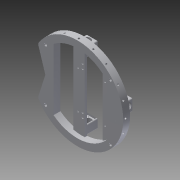
# Autodesk Inventor part: Middle Plate
Saved by Autodesk Inventor 2015 (Build 190159000, 159)
## iProperties
Created: 2015-10-10
Part Number: Middle Plate
Material: ABS Plastic
Document SubType Name: Modeling
Designer: James
Density: 1.06 g/cm^3
Appearance: Smooth - White
Author: James
Autodesk Inventor part; units mm, degrees
(part 1 of 2)
ref_plane "YZ Plane" through (0, 0, 0) normal (1, 0, 0) x (0, 1, 0)
ref_plane "XZ Plane" through (0, 0, 0) normal (0, 1, 0) x (-1, 0, 0)
ref_plane "XY Plane" through (0, 0, 0) normal (0, 0, 1) x (1, 0, 0)
sketch "Sketch1" plane through (0, 0, 0) normal (0, 1, 0) x (-1, 0, 0)
  line L0 (70, 0) -> (70, 48.2183)
  line L1 (70, 0) -> (70, -48.2183)
  arc A0 (70, 48.2183) -> (70, -48.2183) centre (0, 0) ccw
  arc A1 (85, 52.6783) -> (85, -52.6783) centre (0, 0) ccw
  line L2 (85, -52.6783) -> (85, -47.6783)
  line L3 (85, 52.6783) -> (85, 47.6783)
  line L4 (85, -47.6783) -> (70, 0)
  line L5 (70, 0) -> (85, 47.6783)
  dimension "d332" = 5
  dimension "d333" = 5
  constraints: 12 end point, 4 point on circle, 2 centre point, 1 coincident, 1 point on line, 1 vertical
  measures "d332" distance of L2.start L2.end
  measures "d333" distance of L3.start L3.end
extrude "Extrusion1" add sketch "Sketch1" along normal blind 15
sketch "Sketch2" plane through (0, 15, 0) normal (0, 1, 0) x (1, 0, 0)
  circle A0 centre (-69.5802, 56.8899) radius 3
  circle A1 centre (71.6532, 61.1111) radius 3
  circle A2 centre (-69.5802, -56.8899) radius 3
  circle A3 centre (71.6532, -61.1111) radius 3
  point P0 (0, 0)
  dimension "d10" = 6
  dimension "d11" = 6
  constraints: 4 centre point
  measures "d10" diameter of A0
  measures "d11" diameter of A1
extrude "Extrusion2" cut sketch "Sketch2" against normal blind 15
sketch "Sketch3" plane through (0, 15, 0) normal (0, 1, 0) x (1, 0, 0)
  line L0 (-85, 52.6783) -> (-85, -52.6783) projected
  line L1 (-62, 5.2) -> (-62, -5.2)
  line L2 (-62, -5.2) -> (-66.1, -5.2)
  line L3 (-65, 0) -> (-65, 2.9) construction
  line L4 (-65, 0) -> (-65, -2.9) construction
  arc A0 (-66.1, 2.6833) -> (-66.1, -2.6833) centre (-65, 0) ccw
  line L5 (-62, 5.2) -> (-66.1, 5.2)
  line L6 (-66.1, -5.2) -> (-66.1, -2.6833)
  line L7 (-66.1, 2.6833) -> (-66.1, 5.2)
  line L8 (-63.4481, -16.8902) -> (-60.7564, -26.9359)
  line L9 (-60.7564, -26.9359) -> (-64.7167, -27.997)
  arc A1 (-66.757, -20.3823) -> (-65.368, -25.5661) centre (-65, -22.6895) ccw
  line L10 (-63.4481, -16.8902) -> (-67.4084, -17.9514)
  line L11 (-64.7167, -27.997) -> (-65.368, -25.5661)
  line L12 (-60.7564, 26.9359) -> (-63.4481, 16.8902)
  line L13 (-63.4481, 16.8902) -> (-67.4084, 17.9514)
  arc A2 (-65.368, 25.5661) -> (-66.757, 20.3823) centre (-65, 22.6895) ccw
  line L14 (-60.7564, 26.9359) -> (-64.7167, 27.997)
  line L15 (-67.4084, 17.9514) -> (-66.757, 20.3823)
  line L16 (-65.368, 25.5661) -> (-64.7167, 27.997)
  line L17 (-65.0019, 39.3752) -> (-68.5526, 41.4252)
  line L18 (-59.8019, 48.3819) -> (-65.0019, 39.3752)
  line L19 (-59.8019, 48.3819) -> (-63.3526, 50.4319)
  line L20 (-64.611, 48.2524) -> (-63.3526, 50.4319)
  arc A3 (-64.611, 48.2524) -> (-67.2943, 43.6048) centre (-65, 45.3786) ccw
  line L21 (-68.5526, 41.4252) -> (-67.2943, 43.6048)
  line L22 (-65.0019, -39.3752) -> (-59.8019, -48.3819)
  line L23 (-59.8019, -48.3819) -> (-63.3526, -50.4319)
  arc A4 (-67.2943, -43.6048) -> (-64.611, -48.2524) centre (-65, -45.3786) ccw
  line L24 (-65.0019, -39.3752) -> (-68.5526, -41.4252)
  line L25 (-63.3526, -50.4319) -> (-64.611, -48.2524)
  line L26 (-67.2943, -43.6048) -> (-68.5526, -41.4252)
  line L27 (-66.757, -20.3823) -> (-67.4084, -17.9514)
  line L28 (-58.3661, -67.5222) -> (-50.1152, -73.8533)
  line L29 (-50.1152, -73.8533) -> (-52.6111, -77.1061)
  line L30 (-56.0669, -73.0678) -> (-65.1245, -62.2245) construction
  arc A5 (-58.8654, -72.3071) -> (-54.6078, -75.574) centre (-56.0669, -73.0678) ccw
  line L31 (-58.3661, -67.5222) -> (-60.862, -70.775)
  line L32 (-52.6111, -77.1061) -> (-54.6078, -75.574)
  line L33 (-58.8654, -72.3071) -> (-60.862, -70.775)
  line L34 (-34.3361, -82.3826) -> (-24.5197, -85.8175)
  arc A6 (-33.3147, -87.0837) -> (-28.2493, -88.8562) centre (-30.4187, -86.9317) ccw
  line L35 (-34.3361, -82.3826) -> (-35.6902, -86.2525)
  line L36 (-33.3147, -87.0837) -> (-35.6902, -86.2525)
  line L37 (-25.8738, -89.6874) -> (-28.2493, -88.8562)
  line L38 (-24.5197, -85.8175) -> (-25.8738, -89.6874)
  line L39 (-6.8652, -88.9872) -> (3.533, -89.1817)
  arc A7 (-4.4255, -93.1335) -> (0.9401, -93.2339) centre (-1.7222, -92.0839) ccw
  line L40 (-6.8652, -88.9872) -> (-6.9418, -93.0865)
  line L41 (-4.4255, -93.1335) -> (-6.9418, -93.0865)
  line L42 (3.4564, -93.2809) -> (0.9401, -93.2339)
  line L43 (3.533, -89.1817) -> (3.4564, -93.2809)
  line L44 (21.2937, -86.6743) -> (31.2317, -83.6088)
  arc A8 (24.9071, -89.8503) -> (30.0353, -88.2685) centre (27.147, -88.0083) ccw
  line L45 (21.2937, -86.6743) -> (22.5022, -90.5921)
  line L46 (24.9071, -89.8503) -> (22.5022, -90.5921)
  line L47 (32.4402, -87.5267) -> (30.0353, -88.2685)
  line L48 (31.2317, -83.6088) -> (32.4402, -87.5267)
  line L49 (47.3187, -75.6756) -> (55.8005, -69.6574)
  arc A9 (51.7438, -77.563) -> (56.1205, -74.4575) centre (53.2956, -75.1132) ccw
  line L50 (47.3187, -75.6756) -> (49.6912, -79.0194)
  line L51 (51.7438, -77.563) -> (49.6912, -79.0194)
  line L52 (58.1731, -73.0012) -> (56.1205, -74.4575)
  line L53 (55.8005, -69.6574) -> (58.1731, -73.0012)
  line L54 (71.8362, -53.8899) -> (77.5655, -45.2103)
  arc A10 (76.6444, -54.0482) -> (79.6008, -49.5694) centre (77.2046, -51.2028) ccw
  line L55 (71.8362, -53.8899) -> (75.2579, -56.1486)
  line L56 (76.6444, -54.0482) -> (75.2579, -56.1486)
  line L57 (80.9873, -47.469) -> (79.6008, -49.5694)
  line L58 (77.5655, -45.2103) -> (80.9873, -47.469)
  line L59 (83.0102, -32.7896) -> (86.2609, -22.9107)
  arc A11 (87.6914, -31.6805) -> (89.3689, -26.5829) centre (87.4853, -28.7879) ccw
  line L60 (83.0102, -32.7896) -> (86.9048, -34.0711)
  line L61 (87.6914, -31.6805) -> (86.9048, -34.0711)
  line L62 (90.1555, -24.1922) -> (89.3689, -26.5829)
  line L63 (86.2609, -22.9107) -> (90.1555, -24.1922)
  line L64 (89.1, -5.2) -> (89.1, 5.2)
  arc A12 (93.2, -2.6833) -> (93.2, 2.6833) centre (92.1, 0) ccw
  line L65 (89.1, -5.2) -> (93.2, -5.2)
  line L66 (93.2, -2.6833) -> (93.2, -5.2)
  line L67 (93.2, 5.2) -> (93.2, 2.6833)
  line L68 (89.1, 5.2) -> (93.2, 5.2)
  line L69 (86.2609, 22.9107) -> (83.0102, 32.7896)
  arc A13 (89.3689, 26.5829) -> (87.6914, 31.6805) centre (87.4853, 28.7879) ccw
  line L70 (86.2609, 22.9107) -> (90.1555, 24.1922)
  line L71 (89.3689, 26.5829) -> (90.1555, 24.1922)
  line L72 (86.9048, 34.0711) -> (87.6914, 31.6805)
  line L73 (83.0102, 32.7896) -> (86.9048, 34.0711)
  line L74 (77.2547, 44.7549) -> (71.5254, 53.4345)
  arc A14 (79.29, 49.114) -> (76.3336, 53.5927) centre (76.8938, 50.7474) ccw
  line L75 (77.2547, 44.7549) -> (80.6765, 47.0136)
  line L76 (79.29, 49.114) -> (80.6765, 47.0136)
  line L77 (74.9472, 55.6931) -> (76.3336, 53.5927)
  line L78 (71.5254, 53.4345) -> (74.9472, 55.6931)
  line L79 (55.8005, 69.6574) -> (47.3187, 75.6756)
  arc A15 (56.1205, 74.4575) -> (51.7438, 77.563) centre (53.2956, 75.1132) ccw
  line L80 (55.8005, 69.6574) -> (58.1731, 73.0012)
  line L81 (56.1205, 74.4575) -> (58.1731, 73.0012)
  line L82 (49.6912, 79.0194) -> (51.7438, 77.563)
  line L83 (47.3187, 75.6756) -> (49.6912, 79.0194)
  line L84 (31.2317, 83.6088) -> (21.2937, 86.6743)
  arc A16 (30.0353, 88.2685) -> (24.9071, 89.8503) centre (27.147, 88.0083) ccw
  line L85 (31.2317, 83.6088) -> (32.4402, 87.5267)
  line L86 (30.0353, 88.2685) -> (32.4402, 87.5267)
  line L87 (22.5022, 90.5921) -> (24.9071, 89.8503)
  line L88 (21.2937, 86.6743) -> (22.5022, 90.5921)
  line L89 (3.533, 89.1817) -> (-6.8652, 88.9872)
  arc A17 (0.9401, 93.2339) -> (-4.4255, 93.1335) centre (-1.7222, 92.0839) ccw
  line L90 (3.533, 89.1817) -> (3.4564, 93.2809)
  line L91 (0.9401, 93.2339) -> (3.4564, 93.2809)
  line L92 (-6.9418, 93.0865) -> (-4.4255, 93.1335)
  line L93 (-6.8652, 88.9872) -> (-6.9418, 93.0865)
  line L94 (-24.5197, 85.8175) -> (-34.3361, 82.3826)
  arc A18 (-28.2493, 88.8562) -> (-33.3147, 87.0837) centre (-30.4187, 86.9317) ccw
  line L95 (-24.5197, 85.8175) -> (-25.8738, 89.6874)
  line L96 (-28.2493, 88.8562) -> (-25.8738, 89.6874)
  line L97 (-35.6902, 86.2525) -> (-33.3147, 87.0837)
  line L98 (-34.3361, 82.3826) -> (-35.6902, 86.2525)
  line L99 (-50.1152, 73.8533) -> (-58.3661, 67.5222)
  arc A19 (-54.6078, 75.574) -> (-58.8654, 72.3071) centre (-56.0669, 73.0678) ccw
  line L100 (-50.1152, 73.8533) -> (-52.6111, 77.1061)
  line L101 (-54.6078, 75.574) -> (-52.6111, 77.1061)
  line L102 (-60.862, 70.775) -> (-58.8654, 72.3071)
  line L103 (-58.3661, 67.5222) -> (-60.862, 70.775)
  point P0 (0, 0)
  point P1 (-55.6407, -73.3481)
  point P2 (-29.9262, -87.0647)
  point P3 (-1.2128, -92.0563)
  point P4 (27.6222, -87.8228)
  point P5 (53.6891, -74.7885)
  point P6 (87.4853, -28.7879)
  point P7 (92.1, 0)
  point P8 (87.4853, 28.7879)
  point P9 (53.2956, 75.1132)
  point P10 (27.147, 88.0083)
  point P11 (-1.7222, 92.0839)
  point P12 (-30.4187, 86.9317)
  point P13 (-56.0669, 73.0678)
  dimension "d118" = 270
  dimension "d17" = 10.4
  dimension "d18" = 4.1
  dimension "d21" = 180
  dimension "d78" = 10.4
  dimension "d79" = 4.1
  dimension "d81" = 10.4
  dimension "d82" = 4.1
  dimension "d97" = 10.4
  dimension "d98" = 4.1
  dimension "d99" = 10.4
  dimension "d100" = 4.1
  dimension "d114" = 10.4
  dimension "d115" = 4.1
  dimension "d123" = 255
  constraints: 206 end point, 40 point on circle, 20 centre point, 16 coincident, 1 collinear, 152 other
  measures "d17" distance of L1.start L1.end
  measures "d18" distance of L1.end L2.end
  measures "d21" angle of L4 L3
  measures "d78" distance of L10.start L9.start
  measures "d79" distance of L9.start L11.start
  measures "d81" distance of L12.start L13.start
  measures "d82" distance of L13.start L13.end
  measures "d97" distance of L18.start L17.start
  measures "d98" distance of L17.start L17.end
  measures "d99" distance of L24.start L23.start
  measures "d100" distance of L23.start L23.end
  measures "d114" distance of L28.start L28.end
  measures "d115" distance of L28.end L32.start
sketch "Sketch8" plane through (0, 0, 0) normal (0, -1, 0) x (1, 0, 0)
  line L0 (-70, 48.2183) -> (-70, -48.2183)
  arc A0 (-70, -48.2183) -> (-70, 48.2183) centre (0, 0) ccw projected
  line L1 (-52, -48.2183) -> (-52, -67.2384)
  arc A1 (-57, 63.0555) -> (-70, 48.2183) centre (0, 0) ccw
  arc A2 (-70, -48.2183) -> (-52, -67.2384) centre (0, 0) ccw
  line L2 (-52, -48.2183) -> (-52, 67.2384)
  arc A3 (-70, -48.2183) -> (-70, 48.2183) centre (0, 0) ccw projected
  line L3 (-52, -48.2183) -> (63.4566, -48.2183) construction
  dimension "d54" = 18
  dimension "d336" = 90
  constraints: 8 end point, 7 point on circle, 2 centre point, 2 coincident, 2 vertical, 1 horizontal, 1 perpendicular
  measures "d54" distance of L0.end L1.start
  measures "d336" angle of L3 L2
extrude "Extrusion8" add sketch "Sketch8" against normal blind 15 contours A0 L2 L1 L0
sketch "Sketch9" plane through (0, 15, 0) normal (0, 1, 0) x (1, 0, 0)
  circle A0 centre (-8.778, -38.7103) radius 1.6079
  circle A1 centre (-62, -39.9697) radius 1.6079
  circle A2 centre (-62, 34.9127) radius 1.6079
  circle A3 centre (-8.7782, 43.7683) radius 1.6079
  line L0 (-57, 67.2384) -> (-57, -67.2384) projected
  line L1 (-18.7782, -41.2393) -> (-18.7782, -82.8998)
  arc A4 (-52, -67.2384) -> (-52, 67.2384) centre (0, 0) ccw projected
  line L2 (-18.7782, -41.2393) -> (-18.7782, 82.8998)
  line L3 (6.2218, 0) -> (6.2218, -84.772)
  line L4 (6.2218, 84.772) -> (6.2218, 0)
  arc A5 (-18.7782, -82.8998) -> (6.2218, -84.772) centre (0, 0) ccw
  arc A6 (6.2218, 84.772) -> (-18.7782, 82.8998) centre (0, 0) ccw
  circle A7 centre (1.2218, -41.2393) radius 1.65
  circle A8 centre (1.2218, 41.2393) radius 1.65
  point P0 (-8.7782, -84.5455)
  point P1 (-8.7782, 84.5455)
  dimension "d67" = 10.315
  dimension "d215" = 3.3
  dimension "d216" = 3.3
  constraints: 10 point on circle, 8 centre point, 8 end point, 2 coincident, 2 point on line, 1 collinear, 1 vertical alignment
  measures "d67" distance of A0.centre L1.start
  measures "d215" diameter of A7
  measures "d216" diameter of A8
sketch "Sketch10" plane through (0, 15, 0) normal (0, 1, 0) x (1, 0, 0)
  circle A0 centre (-57, -37.4412) radius 1.25
  circle A1 centre (-57, 37.4412) radius 1.25
  point P0 (0, 0)
  dimension "d71" = 2.5
  dimension "d72" = 2.5
  constraints: 2 centre point
  measures "d71" diameter of A0
  measures "d72" diameter of A1
extrude "Extrusion10" cut sketch "Sketch10" against normal blind 10
extrude "Extrusion11" cut sketch "Sketch3" against normal blind 13
sketch "Sketch11" plane through (-62, 15, -5.2) normal (-1, 0, 0) x (0, 0, 1)
  line L0 (72.4384, 0) -> (-62.0384, 0) projected
  line L1 (5.2, 0) -> (5.2, -9.7)
  circle A0 centre (5.2, -9.7) radius 2
  point P0 (5.2, -15)
  dimension "d130" = 9.7
  dimension "d131" = 4
  constraints: 2 end point, 1 centre point, 1 coincident, 1 midpoint, 1 vertical
  measures "d130" distance of L1.start L1.end
  measures "d131" diameter of A0
extrude "Extrusion12" cut sketch "Sketch11" along normal blind 43
sketch "Sketch14" plane through (-63.4481, 2, 16.8902) normal (-0.9659258, 0, 0.258819) x (0.258819, 0, 0.9659258)
  line L0 (0, 13) -> (10.4, 13) projected
  line L1 (5.2, 13) -> (5.2, 3.3)
  circle A0 centre (5.2, 3.3) radius 2
  point P0 (0.1069, -2)
  dimension "d134" = 9.7
  dimension "d135" = 4
  constraints: 2 end point, 1 centre point, 1 coincident, 1 midpoint, 1 vertical
  measures "d134" distance of L1.start L1.end
  measures "d135" diameter of A0
extrude "Extrusion13" cut sketch "Sketch14" along normal blind 67.75
sketch "Sketch15" plane through (-65.0019, 2, 39.3752) normal (-0.8660254, 0, 0.5) x (0.5, 0, 0.8660254)
  line L0 (0, 13) -> (10.4, 13) projected
  line L1 (5.2, 13) -> (5.2, 3.3)
  circle A0 centre (5.2, 3.3) radius 2
  point P0 (-1.599, -2)
  dimension "d138" = 9.7
  dimension "d139" = 4
  constraints: 2 end point, 1 centre point, 1 coincident, 1 midpoint, 1 vertical
  measures "d138" distance of L1.start L1.end
  measures "d139" diameter of A0
extrude "Extrusion14" cut sketch "Sketch15" along normal blind 38.25
sketch "Sketch16" plane through (-60.7564, 2, -26.9359) normal (-0.9659258, 0, -0.258819) x (-0.258819, 0, 0.9659258)
  line L0 (0, 13) -> (10.4, 13) projected
  line L1 (5.2, 13) -> (5.2, 3.3)
  circle A0 centre (5.2, 3.3) radius 2
  point P0 (10.2931, -2)
  dimension "d142" = 9.7
  dimension "d143" = 4
  constraints: 2 end point, 1 centre point, 1 coincident, 1 midpoint, 1 vertical
  measures "d142" distance of L1.start L1.end
  measures "d143" diameter of A0
extrude "Extrusion15" cut sketch "Sketch16" along normal blind 46.75
sketch "Sketch17" plane through (-59.8019, 2, -48.3819) normal (-0.8660254, 0, -0.5) x (-0.5, 0, 0.8660254)
  line L0 (0, 13) -> (10.4, 13) projected
  line L1 (5.2, 13) -> (5.2, 3.3)
  circle A0 centre (5.2, 3.32) radius 2
  point P0 (11.999, -2)
  dimension "d146" = 9.7
  dimension "d147" = 4
  constraints: 2 end point, 1 centre point, 1 midpoint, 1 point on line, 1 vertical
  measures "d146" distance of L1.start L1.end
  measures "d147" diameter of A0
extrude "Extrusion16" cut sketch "Sketch17" along normal blind 31.75
sketch "Sketch18" plane through (-50.1152, 2, -73.8533) normal (-0.6087614, 0, -0.7933533) x (-0.7933533, 0, 0.6087614)
  line L0 (0, 13) -> (10.4, 13) projected
  line L1 (5.2, 13) -> (5.2, 3.3)
  circle A0 centre (5.2, 3.3) radius 2
  point P0 (5.2, -2)
  dimension "d150" = 9.7
  dimension "d151" = 4
  constraints: 2 end point, 1 centre point, 1 coincident, 1 midpoint, 1 vertical
  measures "d150" distance of L1.start L1.end
  measures "d151" diameter of A0
extrude "Extrusion17" cut sketch "Sketch18" along normal blind 15.75
sketch "Sketch19" plane through (-24.5197, 2, -85.8175) normal (-0.3302791, 0, -0.9438833) x (-0.9438833, 0, 0.3302791)
  line L0 (0, 13) -> (10.4, 13) projected
  line L1 (5.2, 13) -> (5.2, 3.3)
  circle A0 centre (5.2, 3.3) radius 2
  point P0 (5.2, -2)
  dimension "d154" = 9.7
  dimension "d155" = 4
  constraints: 2 end point, 1 centre point, 1 coincident, 1 midpoint, 1 vertical
  measures "d154" distance of L1.start L1.end
  measures "d155" diameter of A0
extrude "Extrusion18" cut sketch "Sketch19" along normal blind 15.75
sketch "Sketch20" plane through (3.533, 2, -89.1817) normal (-0.0186989, 0, -0.9998252) x (-0.9998252, 0, 0.0186989)
  line L0 (0, 13) -> (10.4, 13) projected
  line L1 (5.2, 13) -> (5.2, 3.3)
  circle A0 centre (5.2, 3.3) radius 2
  point P0 (5.2, -2)
  dimension "d158" = 9.7
  dimension "d159" = 4
  constraints: 2 end point, 1 centre point, 1 coincident, 1 midpoint, 1 vertical
  measures "d158" distance of L1.start L1.end
  measures "d159" diameter of A0
extrude "Extrusion19" cut sketch "Sketch20" along normal blind 15.75
sketch "Sketch21" plane through (31.2317, 2, -83.6088) normal (0.2947552, 0, -0.9555728) x (-0.9555728, 0, -0.2947552)
  line L0 (0, 13) -> (10.4, 13) projected
  line L1 (5.2, 13) -> (5.2, 3.3)
  circle A0 centre (5.2, 3.3) radius 2
  point P0 (5.2, -2)
  dimension "d162" = 9.7
  dimension "d163" = 4
  constraints: 2 end point, 1 centre point, 1 coincident, 1 midpoint, 1 vertical
  measures "d162" distance of L1.start L1.end
  measures "d163" diameter of A0
extrude "Extrusion20" cut sketch "Sketch21" along normal blind 15.75
sketch "Sketch22" plane through (55.8005, 2, -69.6574) normal (0.5786713, 0, -0.8155609) x (-0.8155609, 0, -0.5786713)
  line L0 (0, 13) -> (10.4, 13) projected
  line L1 (5.2, 13) -> (5.2, 3.3)
  circle A0 centre (5.2, 3.3) radius 2
  point P0 (5.2, -2)
  dimension "d166" = 9.7
  dimension "d167" = 4
  constraints: 2 end point, 1 centre point, 1 coincident, 1 midpoint, 1 vertical
  measures "d166" distance of L1.start L1.end
  measures "d167" diameter of A0
extrude "Extrusion21" cut sketch "Sketch22" along normal blind 15.75
sketch "Sketch23" plane through (77.2547, 2, -44.7549) normal (0.8345733, 0, -0.550897) x (-0.550897, 0, -0.8345733)
  line L0 (0, 13) -> (10.4, 13) projected
  line L1 (5.2, 13) -> (5.2, 3.3)
  circle A0 centre (5.2, 3.3) radius 2
  point P0 (5.2082, -2)
  dimension "d170" = 9.7
  dimension "d171" = 4
  constraints: 2 end point, 1 centre point, 1 coincident, 1 midpoint, 1 vertical
  measures "d170" distance of L1.start L1.end
  measures "d171" diameter of A0
extrude "Extrusion22" cut sketch "Sketch23" along normal blind 15.75
sketch "Sketch24" plane through (86.2609, 2, -22.9107) normal (0.9498941, 0, -0.3125718) x (-0.3125718, 0, -0.9498941)
  line L0 (0, 13) -> (10.4, 13) projected
  line L1 (5.2, 13) -> (5.2, 3.3)
  circle A0 centre (5.2, 3.3) radius 2
  point P0 (5.2, -2)
  dimension "d174" = 9.7
  dimension "d175" = 4
  constraints: 2 end point, 1 centre point, 1 coincident, 1 midpoint, 1 vertical
  measures "d174" distance of L1.start L1.end
  measures "d175" diameter of A0
extrude "Extrusion23" cut sketch "Sketch24" along normal blind 15.75
sketch "Sketch25" plane through (89.1, 15, 5.2) normal (1, 0, 0) x (0, 0, -1)
  line L0 (0, 0) -> (10.4, 0) projected
  line L1 (5.2, 0) -> (5.2, -9.7)
  circle A0 centre (5.2, -9.7) radius 2
  point P0 (5.2, -15)
  dimension "d178" = 9.7
  dimension "d179" = 4
  constraints: 2 end point, 1 centre point, 1 coincident, 1 midpoint, 1 vertical
  measures "d178" distance of L1.start L1.end
  measures "d179" diameter of A0
extrude "Extrusion24" cut sketch "Sketch25" along normal blind 15.75
sketch "Sketch26" plane through (83.0102, 2, 32.7896) normal (0.9498941, 0, 0.3125718) x (0.3125718, 0, -0.9498941)
  line L0 (0, 13) -> (10.4, 13) projected
  line L1 (5.2, 13) -> (5.2, 3.3)
  circle A0 centre (5.2, 3.3) radius 2
  point P0 (5.2, -2)
  dimension "d182" = 9.7
  dimension "d183" = 4
  constraints: 2 end point, 1 centre point, 1 coincident, 1 midpoint, 1 vertical
  measures "d182" distance of L1.start L1.end
  measures "d183" diameter of A0
extrude "Extrusion25" cut sketch "Sketch26" along normal blind 15.75
sketch "Sketch27" plane through (71.8362, 2, 53.8899) normal (0.8345733, 0, 0.550897) x (0.550897, 0, -0.8345733)
  line L0 (0, 13) -> (10.4, 13) projected
  line L1 (5.2, 13) -> (5.2, 3.3)
  circle A0 centre (5.2, 3.3) radius 2
  point P0 (5.4007, -2)
  dimension "d186" = 9.7
  dimension "d187" = 4
  constraints: 2 end point, 1 centre point, 1 coincident, 1 midpoint, 1 vertical
  measures "d186" distance of L1.start L1.end
  measures "d187" diameter of A0
extrude "Extrusion26" cut sketch "Sketch27" along normal blind 15.75
sketch "Sketch28" plane through (47.3187, 2, 75.6756) normal (0.5786713, 0, 0.8155609) x (0.8155609, 0, -0.5786713)
  line L0 (0, 13) -> (10.4, 13) projected
  line L1 (5.2, 13) -> (5.2, 3.3)
  circle A0 centre (5.2, 3.3) radius 2
  point P0 (5.2, -2)
  dimension "d190" = 9.7
  dimension "d191" = 4
  constraints: 2 end point, 1 centre point, 1 coincident, 1 midpoint, 1 vertical
  measures "d190" distance of L1.start L1.end
  measures "d191" diameter of A0
extrude "Extrusion27" cut sketch "Sketch28" along normal blind 15.75
sketch "Sketch29" plane through (21.2937, 2, 86.6743) normal (0.2947552, 0, 0.9555728) x (0.9555728, 0, -0.2947552)
  line L0 (0, 13) -> (10.4, 13) projected
  line L1 (5.2, 13) -> (5.2, 3.3)
  circle A0 centre (5.2, 3.3) radius 2
  point P0 (5.2, -2)
  dimension "d194" = 9.7
  dimension "d195" = 4
  constraints: 2 end point, 1 centre point, 1 coincident, 1 midpoint, 1 vertical
  measures "d194" distance of L1.start L1.end
  measures "d195" diameter of A0
extrude "Extrusion28" cut sketch "Sketch29" along normal blind 15.75
sketch "Sketch30" plane through (-6.8652, 2, 88.9872) normal (-0.0186989, 0, 0.9998252) x (0.9998252, 0, 0.0186989)
  line L0 (0, 13) -> (10.4, 13) projected
  line L1 (5.2, 13) -> (5.2, 3.3)
  circle A0 centre (5.2, 3.3) radius 2
  point P0 (5.2, -2)
  dimension "d198" = 9.7
  dimension "d199" = 4
  constraints: 2 end point, 1 centre point, 1 coincident, 1 midpoint, 1 vertical
  measures "d198" distance of L1.start L1.end
  measures "d199" diameter of A0
extrude "Extrusion29" cut sketch "Sketch30" along normal blind 15.75
sketch "Sketch31" plane through (-34.3361, 2, 82.3826) normal (-0.3302791, 0, 0.9438833) x (0.9438833, 0, 0.3302791)
  line L0 (0, 13) -> (10.4, 13) projected
  line L1 (5.2, 13) -> (5.2, 3.3)
  circle A0 centre (5.2, 3.3) radius 2
  point P0 (5.2, -2)
  dimension "d202" = 9.7
  dimension "d203" = 4
  constraints: 2 end point, 1 centre point, 1 coincident, 1 midpoint, 1 vertical
  measures "d202" distance of L1.start L1.end
  measures "d203" diameter of A0
extrude "Extrusion30" cut sketch "Sketch31" along normal blind 15.75
sketch "Sketch32" plane through (-58.3661, 2, 67.5222) normal (-0.6087614, 0, 0.7933533) x (0.7933533, 0, 0.6087614)
  line L0 (0, 13) -> (10.4, 13) projected
  line L1 (5.2, 13) -> (5.2, 3.3)
  circle A0 centre (5.2, 3.3) radius 2
  point P0 (5.2, -2)
  dimension "d206" = 9.7
  dimension "d207" = 4
  constraints: 2 end point, 1 centre point, 1 coincident, 1 midpoint, 1 vertical
  measures "d206" distance of L1.start L1.end
  measures "d207" diameter of A0
extrude "Extrusion31" cut sketch "Sketch32" along normal blind 15.75
sketch "Sketch33" plane through (0, 15, 0) normal (0, 1, 0) x (1, 0, 0)
  point P0 (0, 0)
extrude "Extrusion33" add sketch "Sketch9" against normal blind 5 contours L2 A4 L4 L3 L1
sketch "Sketch34" plane through (0, 15, 0) normal (0, 1, 0) x (1, 0, 0)
  arc A0 (6.2218, -84.772) -> (6.2218, 84.772) centre (0, 0) ccw projected
  line L0 (45, 0) -> (45, -72.111)
  line L1 (45, 0) -> (45, 72.111)
  arc A1 (45, -72.111) -> (45, 72.111) centre (0, 0) ccw
  constraints: 4 end point, 4 point on circle, 1 centre point, 1 coincident, 1 point on line
extrude "Extrusion34" add sketch "Sketch34" against normal blind 5
sketch "Sketch35" plane through (0, 15, 0) normal (0, 1, 0) x (1, 0, 0)
  arc A0 (-52, -67.2384) -> (-18.7782, -82.8998) centre (0, 0) ccw projected
  line L0 (-52, -67.2384) -> (-52, 67.2384) projected
  arc A1 (-18.7782, 82.8998) -> (-52, 67.2384) centre (0, 0) ccw projected
  line L1 (-18.7782, 82.8998) -> (-18.7782, -82.8998) projected
  circle A2 centre (-8.7782, 43.7683) radius 1.6079 projected
  circle A3 centre (-8.778, -38.7103) radius 1.6079 projected
  circle A4 centre (1.2218, -41.2393) radius 1.65 projected
  circle A5 centre (1.2218, 41.2393) radius 1.65 projected
  line L2 (-28.2493, 88.8562) -> (-25.8738, 89.6874) projected
  line L3 (-25.8738, 89.6874) -> (-24.5197, 85.8175) projected
  line L4 (-24.5197, 85.8175) -> (-34.3361, 82.3826) projected
  line L5 (-34.3361, 82.3826) -> (-35.6902, 86.2525) projected
  line L6 (-35.6902, 86.2525) -> (-33.3147, 87.0837) projected
  arc A6 (-28.2493, 88.8562) -> (-33.3147, 87.0837) centre (-30.4187, 86.9317) ccw projected
  line L7 (30.0353, 88.2685) -> (32.4402, 87.5267) projected
  line L8 (32.4402, 87.5267) -> (31.2317, 83.6088) projected
  line L9 (31.2317, 83.6088) -> (21.2937, 86.6743) projected
  line L10 (21.2937, 86.6743) -> (22.5022, 90.5921) projected
  line L11 (22.5022, 90.5921) -> (24.9071, 89.8503) projected
  arc A7 (30.0353, 88.2685) -> (24.9071, 89.8503) centre (27.147, 88.0083) ccw projected
  line L12 (79.29, 49.114) -> (80.6765, 47.0136) projected
  line L13 (80.6765, 47.0136) -> (77.2547, 44.7549) projected
  line L14 (77.2547, 44.7549) -> (71.5254, 53.4345) projected
  line L15 (71.5254, 53.4345) -> (74.9472, 55.6931) projected
  line L16 (74.9472, 55.6931) -> (76.3336, 53.5927) projected
  arc A8 (79.29, 49.114) -> (76.3336, 53.5927) centre (76.8938, 50.7474) ccw projected
  line L17 (93.2, -2.6833) -> (93.2, -5.2) projected
  line L18 (93.2, -5.2) -> (89.1, -5.2) projected
  line L19 (89.1, -5.2) -> (89.1, 5.2) projected
  line L20 (89.1, 5.2) -> (93.2, 5.2) projected
  line L21 (93.2, 5.2) -> (93.2, 2.6833) projected
  arc A9 (93.2, -2.6833) -> (93.2, 2.6833) centre (92.1, 0) ccw projected
  line L22 (76.6444, -54.0482) -> (75.2579, -56.1486) projected
  line L23 (75.2579, -56.1486) -> (71.8362, -53.8899) projected
  line L24 (71.8362, -53.8899) -> (77.5655, -45.2103) projected
  line L25 (77.5655, -45.2103) -> (80.9873, -47.469) projected
  line L26 (80.9873, -47.469) -> (79.6008, -49.5694) projected
  arc A10 (76.6444, -54.0482) -> (79.6008, -49.5694) centre (77.2046, -51.2028) ccw projected
  line L27 (24.9071, -89.8503) -> (22.5022, -90.5921) projected
  line L28 (22.5022, -90.5921) -> (21.2937, -86.6743) projected
  line L29 (21.2937, -86.6743) -> (31.2317, -83.6088) projected
  line L30 (31.2317, -83.6088) -> (32.4402, -87.5267) projected
  line L31 (32.4402, -87.5267) -> (30.0353, -88.2685) projected
  arc A11 (24.9071, -89.8503) -> (30.0353, -88.2685) centre (27.147, -88.0083) ccw projected
  line L32 (-33.3147, -87.0837) -> (-35.6902, -86.2525) projected
  line L33 (-35.6902, -86.2525) -> (-34.3361, -82.3826) projected
  line L34 (-34.3361, -82.3826) -> (-24.5197, -85.8175) projected
  line L35 (-24.5197, -85.8175) -> (-25.8738, -89.6874) projected
  line L36 (-25.8738, -89.6874) -> (-28.2493, -88.8562) projected
  arc A12 (-33.3147, -87.0837) -> (-28.2493, -88.8562) centre (-30.4187, -86.9317) ccw projected
  line L37 (-68.5526, -41.4252) -> (-65.0019, -39.3752) projected
  line L38 (-65.0019, -39.3752) -> (-59.8019, -48.3819) projected
  line L39 (-59.8019, -48.3819) -> (-63.3526, -50.4319) projected
  line L40 (-63.3526, -50.4319) -> (-64.611, -48.2524) projected
  arc A13 (-67.2943, -43.6048) -> (-64.611, -48.2524) centre (-65, -45.3786) ccw projected
  line L41 (-67.2943, -43.6048) -> (-68.5526, -41.4252) projected
  line L42 (-64.7167, 27.997) -> (-60.7564, 26.9359) projected
  line L43 (-60.7564, 26.9359) -> (-63.4481, 16.8902) projected
  line L44 (-63.4481, 16.8902) -> (-67.4084, 17.9514) projected
  line L45 (-67.4084, 17.9514) -> (-66.757, 20.3823) projected
  arc A14 (-65.368, 25.5661) -> (-66.757, 20.3823) centre (-65, 22.6895) ccw projected
  line L46 (-65.368, 25.5661) -> (-64.7167, 27.997) projected
  line L47 (-66.1, 5.2) -> (-62, 5.2) projected
  line L48 (-62, 5.2) -> (-62, -5.2) projected
  line L49 (-62, -5.2) -> (-66.1, -5.2) projected
  line L50 (-66.1, -5.2) -> (-66.1, -2.6833) projected
  arc A15 (-66.1, 2.6833) -> (-66.1, -2.6833) centre (-65, 0) ccw projected
  line L51 (-66.1, 2.6833) -> (-66.1, 5.2) projected
  line L52 (-67.4084, -17.9514) -> (-63.4481, -16.8902) projected
  line L53 (-63.4481, -16.8902) -> (-60.7564, -26.9359) projected
  line L54 (-60.7564, -26.9359) -> (-64.7167, -27.997) projected
  line L55 (-64.7167, -27.997) -> (-65.368, -25.5661) projected
  arc A16 (-66.757, -20.3823) -> (-65.368, -25.5661) centre (-65, -22.6895) ccw projected
  line L56 (-66.757, -20.3823) -> (-67.4084, -17.9514) projected
  line L57 (-63.3526, 50.4319) -> (-59.8019, 48.3819) projected
  line L58 (-59.8019, 48.3819) -> (-65.0019, 39.3752) projected
  line L59 (-65.0019, 39.3752) -> (-68.5526, 41.4252) projected
  line L60 (-68.5526, 41.4252) -> (-67.2943, 43.6048) projected
  arc A17 (-64.611, 48.2524) -> (-67.2943, 43.6048) centre (-65, 45.3786) ccw projected
  line L61 (-64.611, 48.2524) -> (-63.3526, 50.4319) projected
  line L62 (-60.862, -70.775) -> (-58.3661, -67.5222) projected
  line L63 (-58.3661, -67.5222) -> (-50.1152, -73.8533) projected
  line L64 (-50.1152, -73.8533) -> (-52.6111, -77.1061) projected
  line L65 (-52.6111, -77.1061) -> (-54.6078, -75.574) projected
  arc A18 (-58.8654, -72.3071) -> (-54.6078, -75.574) centre (-56.0669, -73.0678) ccw projected
  line L66 (-58.8654, -72.3071) -> (-60.862, -70.775) projected
  line L67 (-4.4255, -93.1335) -> (-6.9418, -93.0865) projected
  line L68 (-6.9418, -93.0865) -> (-6.8652, -88.9872) projected
  line L69 (-6.8652, -88.9872) -> (3.533, -89.1817) projected
  line L70 (3.533, -89.1817) -> (3.4564, -93.2809) projected
  line L71 (3.4564, -93.2809) -> (0.9401, -93.2339) projected
  arc A19 (-4.4255, -93.1335) -> (0.9401, -93.2339) centre (-1.7222, -92.0839) ccw projected
  line L72 (51.7438, -77.563) -> (49.6912, -79.0194) projected
  line L73 (49.6912, -79.0194) -> (47.3187, -75.6756) projected
  line L74 (47.3187, -75.6756) -> (55.8005, -69.6574) projected
  line L75 (55.8005, -69.6574) -> (58.1731, -73.0012) projected
  line L76 (58.1731, -73.0012) -> (56.1205, -74.4575) projected
  arc A20 (51.7438, -77.563) -> (56.1205, -74.4575) centre (53.2956, -75.1132) ccw projected
  line L77 (87.6914, -31.6805) -> (86.9048, -34.0711) projected
  line L78 (86.9048, -34.0711) -> (83.0102, -32.7896) projected
  line L79 (83.0102, -32.7896) -> (86.2609, -22.9107) projected
  line L80 (86.2609, -22.9107) -> (90.1555, -24.1922) projected
  line L81 (90.1555, -24.1922) -> (89.3689, -26.5829) projected
  arc A21 (87.6914, -31.6805) -> (89.3689, -26.5829) centre (87.4853, -28.7879) ccw projected
  line L82 (89.3689, 26.5829) -> (90.1555, 24.1922) projected
  line L83 (90.1555, 24.1922) -> (86.2609, 22.9107) projected
  line L84 (86.2609, 22.9107) -> (83.0102, 32.7896) projected
  line L85 (83.0102, 32.7896) -> (86.9048, 34.0711) projected
  line L86 (86.9048, 34.0711) -> (87.6914, 31.6805) projected
  arc A22 (89.3689, 26.5829) -> (87.6914, 31.6805) centre (87.4853, 28.7879) ccw projected
  line L87 (56.1205, 74.4575) -> (58.1731, 73.0012) projected
  line L88 (58.1731, 73.0012) -> (55.8005, 69.6574) projected
  line L89 (55.8005, 69.6574) -> (47.3187, 75.6756) projected
  line L90 (47.3187, 75.6756) -> (49.6912, 79.0194) projected
  line L91 (49.6912, 79.0194) -> (51.7438, 77.563) projected
  arc A23 (56.1205, 74.4575) -> (51.7438, 77.563) centre (53.2956, 75.1132) ccw projected
  line L92 (0.9401, 93.2339) -> (3.4564, 93.2809) projected
  line L93 (3.4564, 93.2809) -> (3.533, 89.1817) projected
  line L94 (3.533, 89.1817) -> (-6.8652, 88.9872) projected
  line L95 (-6.8652, 88.9872) -> (-6.9418, 93.0865) projected
  line L96 (-6.9418, 93.0865) -> (-4.4255, 93.1335) projected
  arc A24 (0.9401, 93.2339) -> (-4.4255, 93.1335) centre (-1.7222, 92.0839) ccw projected
  line L97 (-54.6078, 75.574) -> (-52.6111, 77.1061) projected
  line L98 (-52.6111, 77.1061) -> (-50.1152, 73.8533) projected
  line L99 (-50.1152, 73.8533) -> (-58.3661, 67.5222) projected
  line L100 (-58.3661, 67.5222) -> (-60.862, 70.775) projected
  line L101 (-60.862, 70.775) -> (-58.8654, 72.3071) projected
  arc A25 (-54.6078, 75.574) -> (-58.8654, 72.3071) centre (-56.0669, 73.0678) ccw projected
  circle A26 centre (-57, -37.4412) radius 1.25 projected
  circle A27 centre (-57, 37.4412) radius 1.25 projected
  circle A28 centre (-69.5802, -56.8899) radius 3 projected
  circle A29 centre (-69.5802, 56.8899) radius 3 projected
  circle A30 centre (71.6532, 61.1111) radius 3 projected
  circle A31 centre (71.6532, -61.1111) radius 3 projected
  line L102 (6.2218, -84.772) -> (6.2218, 84.772) projected
  arc A32 (45, 72.111) -> (6.2218, 84.772) centre (0, 0) ccw projected
  line L103 (45, 72.111) -> (45, -72.111) projected
  arc A33 (6.2218, -84.772) -> (45, -72.111) centre (0, 0) ccw projected
  arc A34 (-85, -52.6783) -> (-85, 52.6783) centre (0, 0) ccw projected
  circle A35 centre (50, -41.2393) radius 1.65
  circle A36 centre (50, 41.4252) radius 1.65
  line L104 (-85, 52.6783) -> (-85, 47.6783) projected
  line L105 (-85, -47.6783) -> (-85, -52.6783) projected
  line L106 (-70, 0) -> (-85, -47.6783) projected
  line L107 (-85, 47.6783) -> (-70, 0) projected
  dimension "d223" = 3.3
  dimension "d224" = 3.3
  constraints: 2 centre point
  measures "d223" diameter of A35
  measures "d224" diameter of A36
extrude "Extrusion35" cut sketch "Sketch35" against normal blind 5 contours A35 | A36
sketch "Sketch36" plane through (0, 15, 0) normal (0, 1, 0) x (1, 0, 0)
  arc A0 (-85, -52.6783) -> (-85, 52.6783) centre (0, 0) ccw projected
  arc A1 (45, -72.111) -> (45, 72.111) centre (0, 0) ccw projected
  circle A2 centre (75, -20) radius 1.65
  circle A3 centre (75, 20) radius 1.65
  circle A4 centre (50, -41.2393) radius 1.65 projected
  circle A5 centre (50, 41.4252) radius 1.65 projected
  arc A6 (-52, -67.2384) -> (-18.7782, -82.8998) centre (0, 0) ccw projected
  line L0 (-52, -67.2384) -> (-52, 67.2384) projected
  arc A7 (-18.7782, 82.8998) -> (-52, 67.2384) centre (0, 0) ccw projected
  line L1 (-18.7782, 82.8998) -> (-18.7782, -82.8998) projected
  circle A8 centre (-8.7782, 43.7683) radius 1.6079 projected
  circle A9 centre (-8.778, -38.7103) radius 1.6079 projected
  circle A10 centre (1.2218, -41.2393) radius 1.65 projected
  circle A11 centre (1.2218, 41.2393) radius 1.65 projected
  line L2 (-28.2493, 88.8562) -> (-25.8738, 89.6874) projected
  line L3 (-25.8738, 89.6874) -> (-24.5197, 85.8175) projected
  line L4 (-24.5197, 85.8175) -> (-34.3361, 82.3826) projected
  line L5 (-34.3361, 82.3826) -> (-35.6902, 86.2525) projected
  line L6 (-35.6902, 86.2525) -> (-33.3147, 87.0837) projected
  arc A12 (-28.2493, 88.8562) -> (-33.3147, 87.0837) centre (-30.4187, 86.9317) ccw projected
  line L7 (30.0353, 88.2685) -> (32.4402, 87.5267) projected
  line L8 (32.4402, 87.5267) -> (31.2317, 83.6088) projected
  line L9 (31.2317, 83.6088) -> (21.2937, 86.6743) projected
  line L10 (21.2937, 86.6743) -> (22.5022, 90.5921) projected
  line L11 (22.5022, 90.5921) -> (24.9071, 89.8503) projected
  arc A13 (30.0353, 88.2685) -> (24.9071, 89.8503) centre (27.147, 88.0083) ccw projected
  line L12 (79.29, 49.114) -> (80.6765, 47.0136) projected
  line L13 (80.6765, 47.0136) -> (77.2547, 44.7549) projected
  line L14 (77.2547, 44.7549) -> (71.5254, 53.4345) projected
  line L15 (71.5254, 53.4345) -> (74.9472, 55.6931) projected
  line L16 (74.9472, 55.6931) -> (76.3336, 53.5927) projected
  arc A14 (79.29, 49.114) -> (76.3336, 53.5927) centre (76.8938, 50.7474) ccw projected
  line L17 (93.2, -2.6833) -> (93.2, -5.2) projected
  line L18 (93.2, -5.2) -> (89.1, -5.2) projected
  line L19 (89.1, -5.2) -> (89.1, 5.2) projected
  line L20 (89.1, 5.2) -> (93.2, 5.2) projected
  line L21 (93.2, 5.2) -> (93.2, 2.6833) projected
  arc A15 (93.2, -2.6833) -> (93.2, 2.6833) centre (92.1, 0) ccw projected
  line L22 (76.6444, -54.0482) -> (75.2579, -56.1486) projected
  line L23 (75.2579, -56.1486) -> (71.8362, -53.8899) projected
  line L24 (71.8362, -53.8899) -> (77.5655, -45.2103) projected
  line L25 (77.5655, -45.2103) -> (80.9873, -47.469) projected
  line L26 (80.9873, -47.469) -> (79.6008, -49.5694) projected
  arc A16 (76.6444, -54.0482) -> (79.6008, -49.5694) centre (77.2046, -51.2028) ccw projected
  line L27 (24.9071, -89.8503) -> (22.5022, -90.5921) projected
  line L28 (22.5022, -90.5921) -> (21.2937, -86.6743) projected
  line L29 (21.2937, -86.6743) -> (31.2317, -83.6088) projected
  line L30 (31.2317, -83.6088) -> (32.4402, -87.5267) projected
  line L31 (32.4402, -87.5267) -> (30.0353, -88.2685) projected
  arc A17 (24.9071, -89.8503) -> (30.0353, -88.2685) centre (27.147, -88.0083) ccw projected
  line L32 (-33.3147, -87.0837) -> (-35.6902, -86.2525) projected
  line L33 (-35.6902, -86.2525) -> (-34.3361, -82.3826) projected
  line L34 (-34.3361, -82.3826) -> (-24.5197, -85.8175) projected
  line L35 (-24.5197, -85.8175) -> (-25.8738, -89.6874) projected
  line L36 (-25.8738, -89.6874) -> (-28.2493, -88.8562) projected
  arc A18 (-33.3147, -87.0837) -> (-28.2493, -88.8562) centre (-30.4187, -86.9317) ccw projected
  line L37 (-68.5526, -41.4252) -> (-65.0019, -39.3752) projected
  line L38 (-65.0019, -39.3752) -> (-59.8019, -48.3819) projected
  line L39 (-59.8019, -48.3819) -> (-63.3526, -50.4319) projected
  line L40 (-63.3526, -50.4319) -> (-64.611, -48.2524) projected
  arc A19 (-67.2943, -43.6048) -> (-64.611, -48.2524) centre (-65, -45.3786) ccw projected
  line L41 (-67.2943, -43.6048) -> (-68.5526, -41.4252) projected
  line L42 (-64.7167, 27.997) -> (-60.7564, 26.9359) projected
  line L43 (-60.7564, 26.9359) -> (-63.4481, 16.8902) projected
  line L44 (-63.4481, 16.8902) -> (-67.4084, 17.9514) projected
  line L45 (-67.4084, 17.9514) -> (-66.757, 20.3823) projected
  arc A20 (-65.368, 25.5661) -> (-66.757, 20.3823) centre (-65, 22.6895) ccw projected
  line L46 (-65.368, 25.5661) -> (-64.7167, 27.997) projected
  line L47 (-66.1, 5.2) -> (-62, 5.2) projected
  line L48 (-62, 5.2) -> (-62, -5.2) projected
  line L49 (-62, -5.2) -> (-66.1, -5.2) projected
  line L50 (-66.1, -5.2) -> (-66.1, -2.6833) projected
  arc A21 (-66.1, 2.6833) -> (-66.1, -2.6833) centre (-65, 0) ccw projected
  line L51 (-66.1, 2.6833) -> (-66.1, 5.2) projected
  line L52 (-67.4084, -17.9514) -> (-63.4481, -16.8902) projected
  line L53 (-63.4481, -16.8902) -> (-60.7564, -26.9359) projected
  line L54 (-60.7564, -26.9359) -> (-64.7167, -27.997) projected
  line L55 (-64.7167, -27.997) -> (-65.368, -25.5661) projected
  arc A22 (-66.757, -20.3823) -> (-65.368, -25.5661) centre (-65, -22.6895) ccw projected
  line L56 (-66.757, -20.3823) -> (-67.4084, -17.9514) projected
  line L57 (-63.3526, 50.4319) -> (-59.8019, 48.3819) projected
  line L58 (-59.8019, 48.3819) -> (-65.0019, 39.3752) projected
  line L59 (-65.0019, 39.3752) -> (-68.5526, 41.4252) projected
  line L60 (-68.5526, 41.4252) -> (-67.2943, 43.6048) projected
  arc A23 (-64.611, 48.2524) -> (-67.2943, 43.6048) centre (-65, 45.3786) ccw projected
  line L61 (-64.611, 48.2524) -> (-63.3526, 50.4319) projected
  line L62 (-60.862, -70.775) -> (-58.3661, -67.5222) projected
  line L63 (-58.3661, -67.5222) -> (-50.1152, -73.8533) projected
  line L64 (-50.1152, -73.8533) -> (-52.6111, -77.1061) projected
  line L65 (-52.6111, -77.1061) -> (-54.6078, -75.574) projected
  arc A24 (-58.8654, -72.3071) -> (-54.6078, -75.574) centre (-56.0669, -73.0678) ccw projected
  line L66 (-58.8654, -72.3071) -> (-60.862, -70.775) projected
  line L67 (-4.4255, -93.1335) -> (-6.9418, -93.0865) projected
  line L68 (-6.9418, -93.0865) -> (-6.8652, -88.9872) projected
  line L69 (-6.8652, -88.9872) -> (3.533, -89.1817) projected
  line L70 (3.533, -89.1817) -> (3.4564, -93.2809) projected
  line L71 (3.4564, -93.2809) -> (0.9401, -93.2339) projected
  arc A25 (-4.4255, -93.1335) -> (0.9401, -93.2339) centre (-1.7222, -92.0839) ccw projected
  line L72 (51.7438, -77.563) -> (49.6912, -79.0194) projected
  line L73 (49.6912, -79.0194) -> (47.3187, -75.6756) projected
  line L74 (47.3187, -75.6756) -> (55.8005, -69.6574) projected
  line L75 (55.8005, -69.6574) -> (58.1731, -73.0012) projected
  line L76 (58.1731, -73.0012) -> (56.1205, -74.4575) projected
  arc A26 (51.7438, -77.563) -> (56.1205, -74.4575) centre (53.2956, -75.1132) ccw projected
  line L77 (87.6914, -31.6805) -> (86.9048, -34.0711) projected
  line L78 (86.9048, -34.0711) -> (83.0102, -32.7896) projected
  line L79 (83.0102, -32.7896) -> (86.2609, -22.9107) projected
  line L80 (86.2609, -22.9107) -> (90.1555, -24.1922) projected
  line L81 (90.1555, -24.1922) -> (89.3689, -26.5829) projected
  arc A27 (87.6914, -31.6805) -> (89.3689, -26.5829) centre (87.4853, -28.7879) ccw projected
  line L82 (89.3689, 26.5829) -> (90.1555, 24.1922) projected
  line L83 (90.1555, 24.1922) -> (86.2609, 22.9107) projected
  line L84 (86.2609, 22.9107) -> (83.0102, 32.7896) projected
  line L85 (83.0102, 32.7896) -> (86.9048, 34.0711) projected
  line L86 (86.9048, 34.0711) -> (87.6914, 31.6805) projected
  arc A28 (89.3689, 26.5829) -> (87.6914, 31.6805) centre (87.4853, 28.7879) ccw projected
  line L87 (56.1205, 74.4575) -> (58.1731, 73.0012) projected
  line L88 (58.1731, 73.0012) -> (55.8005, 69.6574) projected
  line L89 (55.8005, 69.6574) -> (47.3187, 75.6756) projected
  line L90 (47.3187, 75.6756) -> (49.6912, 79.0194) projected
  line L91 (49.6912, 79.0194) -> (51.7438, 77.563) projected
  arc A29 (56.1205, 74.4575) -> (51.7438, 77.563) centre (53.2956, 75.1132) ccw projected
  line L92 (0.9401, 93.2339) -> (3.4564, 93.2809) projected
  line L93 (3.4564, 93.2809) -> (3.533, 89.1817) projected
  line L94 (3.533, 89.1817) -> (-6.8652, 88.9872) projected
  line L95 (-6.8652, 88.9872) -> (-6.9418, 93.0865) projected
  line L96 (-6.9418, 93.0865) -> (-4.4255, 93.1335) projected
  arc A30 (0.9401, 93.2339) -> (-4.4255, 93.1335) centre (-1.7222, 92.0839) ccw projected
  line L97 (-54.6078, 75.574) -> (-52.6111, 77.1061) projected
  line L98 (-52.6111, 77.1061) -> (-50.1152, 73.8533) projected
  line L99 (-50.1152, 73.8533) -> (-58.3661, 67.5222) projected
  line L100 (-58.3661, 67.5222) -> (-60.862, 70.775) projected
  line L101 (-60.862, 70.775) -> (-58.8654, 72.3071) projected
  arc A31 (-54.6078, 75.574) -> (-58.8654, 72.3071) centre (-56.0669, 73.0678) ccw projected
  circle A32 centre (-57, -37.4412) radius 1.25 projected
  circle A33 centre (-57, 37.4412) radius 1.25 projected
  circle A34 centre (-69.5802, -56.8899) radius 3 projected
  circle A35 centre (-69.5802, 56.8899) radius 3 projected
  circle A36 centre (71.6532, 61.1111) radius 3 projected
  circle A37 centre (71.6532, -61.1111) radius 3 projected
  line L102 (6.2218, -84.772) -> (6.2218, 84.772) projected
  arc A38 (45, 72.111) -> (6.2218, 84.772) centre (0, 0) ccw projected
  line L103 (45, 72.111) -> (45, -72.111) projected
  arc A39 (6.2218, -84.772) -> (45, -72.111) centre (0, 0) ccw projected
  arc A40 (-85, -52.6783) -> (-85, 52.6783) centre (0, 0) ccw projected
  circle A41 centre (1.2218, -41.2393) radius 1.65 projected
  circle A42 centre (1.2218, 41.2393) radius 1.65 projected
  circle A43 centre (1.2218, -51.2393) radius 1.65
  circle A44 centre (1.2218, 51.2393) radius 1.65
  line L104 (-85, 52.6783) -> (-85, 47.6783) projected
  line L105 (-85, -47.6783) -> (-85, -52.6783) projected
  line L106 (-70, 0) -> (-85, -47.6783) projected
  line L107 (-85, 47.6783) -> (-70, 0) projected
  dimension "d231" = 3.3
  dimension "d232" = 3.3
  dimension "d240" = 3.3
  dimension "d242" = 3.3
  constraints: 4 centre point
  measures "d231" diameter of A2
  measures "d232" diameter of A3
  measures "d240" diameter of A43
  measures "d242" diameter of A44
extrude "Extrusion36" cut sketch "Sketch36" against normal blind 5 contours A2 | A3 | A43 | A44